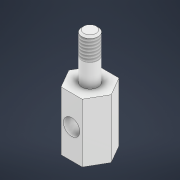
# Autodesk Inventor part: 18102021-002-04
Saved by Autodesk Inventor 2021 (Build 250183000, 183)
## iProperties
Created: 2021-10-15
Part Number: 18102021-002-04
Material: ABS Plastic
Document SubType Name: Modeling
Designer: DuctopwH
Density: 1.06 g/cm^3
Appearance: Smooth - White
Author: DuctopwH
Autodesk Inventor part; units mm, degrees
ref_plane "YZ Plane" through (0, 0, 0) normal (1, 0, 0) x (0, 1, 0)
ref_plane "XZ Plane" through (0, 0, 0) normal (0, 1, 0) x (-1, 0, 0)
ref_plane "XY Plane" through (0, 0, 0) normal (0, 0, 1) x (1, 0, 0)
sketch "Sketch1" plane through (0, 0, 0) normal (0, 1, 0) x (-1, 0, 0)
  line L0 (-1.6252, -2.815) -> (-3.2505, 0)
  line L1 (-3.2505, 0) -> (-1.6252, 2.815)
  line L2 (-1.6252, 2.815) -> (1.6252, 2.815)
  line L3 (1.6252, 2.815) -> (3.2505, 0)
  line L4 (3.2505, 0) -> (1.6252, -2.815)
  line L5 (1.6252, -2.815) -> (-1.6252, -2.815)
  point P0 (0, 0)
  point P1 (0, 0)
  dimension "d0" = 5.63
  constraints: 12 end point, 1 coincident, 1 horizontal, 13 other
  measures "d0" distance between parallel lines of L0 L3
extrude "Extrusion1" add sketch "Sketch1" along normal blind 9
sketch "Sketch2" plane through (0, 9, 0) normal (0, 1, 0) x (1, 0, 0)
  circle A0 centre (0, 0) radius 1.25
  dimension "d3" = 2.5
  constraints: 1 centre point, 1 coincident
  measures "d3" diameter of A0
extrude "Extrusion2" add sketch "Sketch2" along normal blind 7
thread "Thread1" size "M2.5x0.45" class "6g" standard "ANSI Metric M Profile" length 3.5
chamfer "Chamfer1" distance 0.3 angle 45 1 edges at (-1.25, 16, 0)
sketch "Sketch3" plane through (-1.6252, 0, 2.815) normal (0, 0, 1) x (1, 0, 0)
  circle A0 centre (1.6252, 4.5) radius 1.25
  line L0 (0, 0) -> (3.2505, 0) projected
  point P0 (1.6252, 0)
  point P1 (1.6252, 0)
  dimension "d11" = 2.5
  dimension "d12" = 4.5
  constraints: 1 centre point, 1 midpoint, 1 vertical alignment
  measures "d11" diameter of A0
  measures "d12" distance of point (1.625, 0) A0.centre
extrude "Extrusion3" cut sketch "Sketch3" against normal through all
sketch "Sketch4" plane through (0, 0, 0) normal (0, -1, 0) x (1, 0, 0)
  circle A0 centre (0, 0) radius 1.25
  dimension "d15" = 2.5
  constraints: 1 centre point, 1 coincident
  measures "d15" diameter of A0
extrude "Extrusion4" cut sketch "Sketch4" against normal blind 4.5
body "Solid1"
